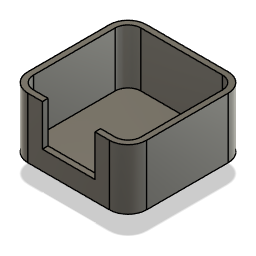
Z-Axis Mount (+-0.2mm) (Autodesk Fusion 360 design; units mm, degrees)
Autodesk Fusion 360 part; units mm, degrees
sketch "Sketch1" plane through (0, 0, 0) normal (0, 1, 0) x (1, 0, 0)
  line L0 (-15.85, 20.85) -> (15.85, 20.85)
  line L1 (20.85, 15.85) -> (20.85, -15.85)
  line L2 (15.85, -20.85) -> (-15.85, -20.85)
  line L3 (-20.85, -15.85) -> (-20.85, 15.85)
  line L4 (-20.85, 20.85) -> (20.85, -20.85) construction
  line L5 (20.85, 20.85) -> (-20.85, -20.85) construction
  arc A0 (-15.85, 20.85) -> (-20.85, 15.85) centre (-15.85, 15.85) ccw
  arc A1 (20.85, 15.85) -> (15.85, 20.85) centre (15.85, 15.85) ccw
  arc A2 (15.85, -20.85) -> (20.85, -15.85) centre (15.85, -15.85) ccw
  arc A3 (-20.85, -15.85) -> (-15.85, -20.85) centre (-15.85, -15.85) ccw
  arc A4 (23.05, 15.85) -> (15.85, 23.05) centre (15.85, 15.85) ccw
  line L6 (-15.85, 23.05) -> (15.85, 23.05)
  arc A5 (-15.85, 23.05) -> (-23.05, 15.85) centre (-15.85, 15.85) ccw
  line L7 (-23.05, -15.85) -> (-23.05, 15.85)
  arc A6 (-23.05, -15.85) -> (-15.85, -23.05) centre (-15.85, -15.85) ccw
  line L8 (15.85, -23.05) -> (-15.85, -23.05)
  arc A7 (15.85, -23.05) -> (23.05, -15.85) centre (15.85, -15.85) ccw
  line L9 (23.05, 15.85) -> (23.05, -15.85)
  dimension "d1" = 41.7
  dimension "d2" = 41.7
  dimension "d3" = 5
  dimension "d4" = -2.2
  constraint horizontal L0
  constraint perpendicular L0 L1
  constraint parallel L0 L2
  constraint parallel L1 L3
  constraint coincident L4 origin
  constraint coincident L5 origin
  constraint coincident L4.start L3
  constraint coincident L4.start L0
  constraint tangent L3 A0
  constraint tangent L0 A0
  constraint coincident L5.start L0
  constraint coincident L5.start L1
  constraint tangent L0 A1
  constraint tangent L1 A1
  constraint equal A0 A1
  constraint coincident L4.end L1
  constraint coincident L4.end L2
  constraint tangent L1 A2
  constraint tangent L2 A2
  constraint equal A0 A2
  constraint coincident L5.end L2
  constraint coincident L5.end L3
  constraint tangent L2 A3
  constraint tangent L3 A3
  constraint equal A0 A3
  measures "d1" distance of L4.end L5.end
  measures "d2" distance of L5.start L4.end
  measures "d3" radius of A0
extrude "Extrude1" add sketch "Sketch1" along normal blind 2.2 contours L0 L1 L2 L3 A0 A1 A2 A3 | A4 L6 A5 L7 A6 L8 A7 L9
extrude "Extrude2" add sketch "Sketch1" along normal blind 23.4
sketch "Sketch2" plane through (0, 0, 23.05) normal (0, 0, 1) x (1, 0, 0)
  line L0 (-15.85, 0) -> (15.85, 0)
  line L1 (15.85, 0) -> (15.85, 23.4)
  line L2 (15.85, 23.4) -> (-15.85, 23.4)
  line L3 (-15.85, 23.4) -> (-15.85, 0)
  line L4 (10.2, 7.4) -> (-10.2, 7.4)
  line L5 (-10.2, 7.4) -> (-10.2, 23.4)
  line L6 (-10.2, 23.4) -> (10.2, 23.4)
  line L7 (10.2, 23.4) -> (10.2, 7.4)
  line L8 (-23.05, 0) -> (-23.05, 23.4)
  line L9 (23.05, 0) -> (23.05, 23.4)
  dimension "d9" = 7.4
  dimension "d10" = 20.4
  dimension "d11" = 16
  dimension "d13" = 12.85
  dimension "d14" = 12.85
  constraint horizontal L4
  constraint vertical L5
  constraint horizontal L6
  constraint vertical L7
  measures "d9" distance of L0 L4
  measures "d10" distance of L5 L7
  measures "d11" distance of L4 L6
  measures "d13" distance of L5 L8
  measures "d14" distance of L7 L9
extrude "Extrude3" cut sketch "Sketch2" against normal blind 2.2 contours L2 L4 L5 L6 L7
ref_plane "WorkPlane1" through (0, 11.7, 0) normal (1, 0, 0) x (0, 0, -1)
sketch "Sketch3" plane through (0, 0, 0) normal (1, 0, 0) x (0, 0, -1)
  line L0 (5.2, 0) -> (12.4125, -7.2125)
  line L1 (5.2, 0) -> (14.8, 0) construction
  line L2 (5.2, 0) -> (-5.2, 0)
  line L3 (-5.2, 0) -> (-12.4125, -7.2125)
  line L4 (12.4125, -7.2125) -> (-12.4125, -7.2125)
  point P0 (23.05, 0)
  point P1 (-23.05, 0)
  dimension "d18" = 10.2
  dimension "d19" = 45
  dimension "d20" = 45
  dimension "d21" = 10.2
  dimension "d22" = 10.4
  dimension "d23" = 17.85
  dimension "d24" = 17.85
  constraint horizontal L1
  constraint parallel L1 L2
  measures "d18" distance of L0.start L0.end
  measures "d19" angle of L0 L1
  measures "d20" angle of L2 L3
  measures "d21" distance of L2.end L3.end
  measures "d22" distance of L0.start L2.end
  measures "d23" distance of L0.start P0
  measures "d24" distance of L2.end P1
extrude "Extrude4" add sketch "Sketch3" along normal mid plane 10.4
equation "d1 = 41.3 mm + 0.2 mm + 0.2 mm"
equation "d2 = 41.3 mm + 0.2 mm + 0.2 mm"
equation "d4 = -( 2 mm + 0.2 mm )"
equation "d5 = 2 mm + 0.2 mm"
equation "d7 = 2 mm + 0.2 mm + 21 mm + 0.2 mm"
equation "d9 = 2 mm + 0.2 mm + 5 mm + 0.2 mm"
equation "d10 = 20 mm + 0.2 mm + 0.2 mm"
equation "d11 = ( 2 mm + 0.2 mm + 21 mm + 0.2 mm ) - ( 2 mm + 0.2 mm + 5 mm + 0.2 mm )"
equation "d13 = ( ( 41.3 mm + 0.2 mm + 0.2 mm + 2 mm + 0.2 mm + 2 mm + 0.2 mm ) - ( 20 mm + 0.2 mm + 0.2 mm ) ) / 2"
equation "d15 = -( 2 mm + 0.2 mm )"
equation "d17 = -( ( ( 41.3 + 0.2 + 0.2 + 2 + 0.2 + 2 + 0.2 ) / 2 ) * 1 mm )"
equation "d18 = 10 mm + 0.2 mm"
equation "d21 = 10 mm + 0.2 mm"
equation "d22 = 10 mm + 0.2 mm + 0.2 mm"
equation "d23 = ( ( ( 41.3 + 0.2 + 0.2 + 2 + 0.2 + 2 + 0.2 ) / 2 ) * 1 mm ) - ( 5 mm + 0.2 mm )"
equation "d25 = 5 mm + 0.2 mm"
